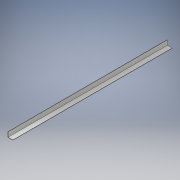
# Autodesk Inventor part: 32-LBracketVersaFrame-1111-2018
Saved by Autodesk Inventor 2017 (Build 210142000, 142)
## iProperties
Created: 2018-04-10
Part Number: 32-LBracketVersaFrame-1111-2018
Material: Generic
Document SubType Name: Modeling
Designer: Phyllis
Density: 1 g/cm^3
Appearance: Aluminum - Polished
Author: Phyllis
Autodesk Inventor part; units mm, degrees
ref_plane "YZ Plane" through (0, 0, 0) normal (1, 0, 0) x (0, 1, 0)
ref_plane "XZ Plane" through (0, 0, 0) normal (0, 1, 0) x (-1, 0, 0)
ref_plane "XY Plane" through (0, 0, 0) normal (0, 0, 1) x (1, 0, 0)
sketch "Sketch1" plane through (0, 0, 0) normal (0, 0, 1) x (1, 0, 0)
  line L0 (0, 0) -> (25.4, 0)
  line L1 (25.4, 0) -> (25.4, 1.5875)
  line L2 (25.4, 1.5875) -> (1.5875, 1.5875)
  line L3 (0, 0) -> (0, 25.4)
  line L4 (0, 25.4) -> (1.5875, 25.4)
  line L5 (1.5875, 1.5875) -> (1.5875, 25.4)
  dimension "d0" = 25.4
  dimension "d1" = 1.5875
  dimension "d2" = 25.4
  dimension "d3" = 1.5875
  constraints: 12 end point, 2 horizontal, 2 perpendicular, 2 vertical
  measures "d0" distance of L0.start L0.end
  measures "d1" distance of L0.end L1.end
  measures "d2" distance of L0.start L3.end
  measures "d3" distance of L3.end L4.end
extrude "Extrusion1" add sketch "Sketch1" along normal blind 1498.6
sketch "Sketch2" plane through (0, 0, 1498.6) normal (0, 0, 1) x (1, 0, 0)
  line L0 (0, 0) -> (25.4, 0) projected
  line L1 (25.4, 0) -> (25.4, 1.5875) projected
  line L2 (25.4, 1.5875) -> (1.5875, 1.5875) projected
  line L3 (1.5875, 1.5875) -> (1.5875, 25.4) projected
  line L4 (1.5875, 25.4) -> (0, 25.4) projected
  line L5 (0, 25.4) -> (0, 0) projected
extrude "Extrusion2" cut sketch "Sketch2" against normal blind 812.8 keep common part
body "Solid1"
